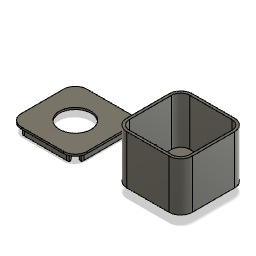
Case Button v3 (Autodesk Fusion 360 design; units mm, degrees)
Autodesk Fusion 360 part; units mm, degrees
sketch "Sketch1" plane through (0, 0, 0) normal (0, 1, 0) x (1, 0, 0)
  line L0 (5, 0) -> (23, 0)
  line L1 (28, -5) -> (28, -23)
  line L2 (23, -28) -> (5, -28)
  line L3 (0, -23) -> (0, -5)
  arc A0 (5, 0) -> (0, -5) centre (5, -5) ccw
  arc A1 (28, -5) -> (23, 0) centre (23, -5) ccw
  arc A2 (23, -28) -> (28, -23) centre (23, -23) ccw
  arc A3 (0, -23) -> (5, -28) centre (5, -23) ccw
  point P0 (28, 0)
  point P1 (0, -28)
  dimension "d1" = 28
  dimension "d2" = 28
  dimension "d3" = 5
  constraint horizontal L0
  constraint vertical L1
  constraint horizontal L2
  constraint vertical L3
  constraint coincident origin L0
  constraint coincident origin L3
  constraint tangent L0 A0
  constraint tangent L3 A0
  constraint coincident P0 L0
  constraint coincident P0 L1
  constraint tangent L0 A1
  constraint tangent L1 A1
  constraint equal A0 A1
  constraint tangent L1 A2
  constraint tangent L2 A2
  constraint equal A0 A2
  constraint coincident P1 L2
  constraint coincident P1 L3
  constraint tangent L2 A3
  constraint tangent L3 A3
  constraint equal A0 A3
  measures "d1" distance of origin P0
  measures "d2" distance of origin P1
  measures "d3" radius of A0
extrude "Extrude1" add sketch "Sketch1" along normal blind 0.8 makes body 1
sketch "Sketch2" plane through (0, 0.8, 0) normal (0, 1, 0) x (-1, 0, 0)
  arc A0 (-5, 0) -> (0, 5) centre (-5, 5) ccw
  line L0 (0, 5) -> (0, 23)
  arc A1 (0, 23) -> (-5, 28) centre (-5, 23) ccw
  line L1 (-5, 28) -> (-23, 28)
  arc A2 (-23, 28) -> (-28, 23) centre (-23, 23) ccw
  line L2 (-28, 23) -> (-28, 5)
  arc A3 (-28, 5) -> (-23, 0) centre (-23, 5) ccw
  line L3 (-23, 0) -> (-5, 0)
  line L4 (0, 14) -> (-28, 14)
  line L5 (-14, 0) -> (-14, 28)
  circle A4 centre (-14, 14) radius 6.75
  dimension "d6" = 13.5
  constraint midpoint L0 L4.start
  constraint midpoint L2 L4.end
  constraint midpoint L3 L5.start
  constraint midpoint L1 L5.end
  constraint midpoint L4 A4.centre
  measures "d6" diameter of A4
extrude "Extrude2" cut sketch "Sketch2" against normal blind 10 contours L4 L5 A4 | L4 L5 A4 | L4 L5 A4 | L4 L5 A4 bodies 1
sketch "Sketch3" plane through (0, 0, 0) normal (0, -1, 0) x (1, 0, 0)
  circle A0 centre (14, 14) radius 6.75
  arc A1 (0, 5) -> (5, 0) centre (5, 5) ccw
  line L0 (5, 0) -> (23, 0)
  arc A2 (23, 0) -> (28, 5) centre (23, 5) ccw
  line L1 (28, 5) -> (28, 23)
  arc A3 (28, 23) -> (23, 28) centre (23, 23) ccw
  line L2 (23, 28) -> (5, 28)
  arc A4 (5, 28) -> (0, 23) centre (5, 23) ccw
  line L3 (0, 23) -> (0, 5)
  arc A5 (5, 26.7) -> (1.3, 23) centre (5, 23) ccw
  line L4 (1.3, 23) -> (1.3, 5)
  arc A6 (1.3, 5) -> (5, 1.3) centre (5, 5) ccw
  line L5 (5, 1.3) -> (23, 1.3)
  arc A7 (23, 1.3) -> (26.7, 5) centre (23, 5) ccw
  line L6 (26.7, 5) -> (26.7, 23)
  arc A8 (26.7, 23) -> (23, 26.7) centre (23, 23) ccw
  line L7 (23, 26.7) -> (5, 26.7)
  arc A9 (5, 25.9) -> (2.1, 23) centre (5, 23) ccw
  line L8 (2.1, 23) -> (2.1, 5)
  arc A10 (2.1, 5) -> (5, 2.1) centre (5, 5) ccw
  line L9 (5, 2.1) -> (23, 2.1)
  arc A11 (23, 2.1) -> (25.9, 5) centre (23, 5) ccw
  line L10 (25.9, 5) -> (25.9, 23)
  arc A12 (25.9, 23) -> (23, 25.9) centre (23, 23) ccw
  line L11 (23, 25.9) -> (5, 25.9)
  dimension "d9" = -1.3
  dimension "d10" = -2.1
extrude "Extrude3" add sketch "Sketch3" along normal blind 3.2 contours A5 L4 A6 L5 A7 L6 A8 L7 bodies 1
sketch "Sketch4" plane through (0, 0.8, 0) normal (0, 1, 0) x (-1, 0, 0)
  circle A0 centre (-14, 14) radius 6.75
  arc A1 (-5, 0) -> (0, 5) centre (-5, 5) ccw
  line L0 (0, 5) -> (0, 23)
  arc A2 (0, 23) -> (-5, 28) centre (-5, 23) ccw
  line L1 (-5, 28) -> (-23, 28)
  arc A3 (-23, 28) -> (-28, 23) centre (-23, 23) ccw
  line L2 (-28, 23) -> (-28, 5)
  arc A4 (-28, 5) -> (-23, 0) centre (-23, 5) ccw
  line L3 (-23, 0) -> (-5, 0)
  line L4 (-50, 0) -> (-68, 0)
  line L5 (-73, 5) -> (-73, 23)
  line L6 (-68, 28) -> (-50, 28)
  line L7 (-45, 23) -> (-45, 5)
  arc A5 (-50, 0) -> (-45, 5) centre (-50, 5) ccw
  arc A6 (-73, 5) -> (-68, 0) centre (-68, 5) ccw
  arc A7 (-68, 28) -> (-73, 23) centre (-68, 23) ccw
  arc A8 (-45, 23) -> (-50, 28) centre (-50, 23) ccw
  point P0 (-45, 0)
  point P1 (-73, 0)
  point P2 (-45, 28)
  dimension "d13" = 28
  dimension "d14" = 28
  dimension "d15" = 5
  constraint horizontal L4
  constraint vertical L5
  constraint horizontal L6
  constraint vertical L7
  constraint coincident P0 L4
  constraint coincident P0 L7
  constraint tangent L4 A5
  constraint tangent L7 A5
  constraint coincident P1 L4
  constraint coincident P1 L5
  constraint tangent L4 A6
  constraint tangent L5 A6
  constraint equal A5 A6
  constraint tangent L5 A7
  constraint tangent L6 A7
  constraint equal A5 A7
  constraint coincident P2 L6
  constraint coincident P2 L7
  constraint tangent L6 A8
  constraint tangent L7 A8
  constraint equal A5 A8
  measures "d13" distance of P0 P1
  measures "d14" distance of P0 P2
  measures "d15" radius of A5
extrude "Extrude4" add sketch "Sketch4" along normal blind 0.8 separate body contours L4 L5 L6 L7 A5 A6 A7 A8 makes body 2
sketch "Sketch5" plane through (0, 1.6, 0) normal (0, 1, 0) x (-1, 0, 0)
  arc A0 (-50, 0) -> (-45, 5) centre (-50, 5) ccw
  line L0 (-45, 5) -> (-45, 23)
  arc A1 (-45, 23) -> (-50, 28) centre (-50, 23) ccw
  line L1 (-50, 28) -> (-68, 28)
  arc A2 (-68, 28) -> (-73, 23) centre (-68, 23) ccw
  line L2 (-73, 23) -> (-73, 5)
  arc A3 (-73, 5) -> (-68, 0) centre (-68, 5) ccw
  line L3 (-68, 0) -> (-50, 0)
  arc A4 (-46.1, 23) -> (-50, 26.9) centre (-50, 23) ccw
  line L4 (-50, 26.9) -> (-68, 26.9)
  arc A5 (-68, 26.9) -> (-71.9, 23) centre (-68, 23) ccw
  line L5 (-71.9, 23) -> (-71.9, 5)
  arc A6 (-71.9, 5) -> (-68, 1.1) centre (-68, 5) ccw
  line L6 (-68, 1.1) -> (-50, 1.1)
  arc A7 (-50, 1.1) -> (-46.1, 5) centre (-50, 5) ccw
  line L7 (-46.1, 5) -> (-46.1, 23)
  dimension "d18" = -1.1
extrude "Extrude5" add sketch "Sketch5" along normal blind 20 bodies 2
sketch "Sketch6" plane through (0, -3.2, 0) normal (0, -1, 0) x (1, 0, 0)
  line L0 (5, 25.9) -> (23, 25.9)
  arc A0 (25.9, 23) -> (23, 25.9) centre (23, 23) ccw
  line L1 (25.9, 23) -> (25.9, 5)
  arc A1 (23, 2.1) -> (25.9, 5) centre (23, 5) ccw
  line L2 (23, 2.1) -> (5, 2.1)
  arc A2 (2.1, 5) -> (5, 2.1) centre (5, 5) ccw
  line L3 (2.1, 5) -> (2.1, 23)
  arc A3 (5, 25.9) -> (2.1, 23) centre (5, 23) ccw
  line L4 (23, 26.7) -> (5, 26.7)
  arc A4 (5, 26.7) -> (1.3, 23) centre (5, 23) ccw
  line L5 (1.3, 23) -> (1.3, 5)
  arc A5 (1.3, 5) -> (5, 1.3) centre (5, 5) ccw
  line L6 (5, 1.3) -> (23, 1.3)
  arc A6 (23, 1.3) -> (26.7, 5) centre (23, 5) ccw
  line L7 (26.7, 5) -> (26.7, 23)
  arc A7 (26.7, 23) -> (23, 26.7) centre (23, 23) ccw
  line L8 (14, 25.9) -> (14, 1.3)
  line L9 (2.1, 14) -> (26.7, 14)
  line L10 (28.4207, 4.0183) -> (-0.4207, 4.0183)
  line L11 (-0.4207, 4.0183) -> (-0.4207, 23.9817)
  line L12 (-0.4207, 23.9817) -> (28.4207, 23.9817)
  line L13 (28.4207, 23.9817) -> (28.4207, 4.0183)
  line L14 (28.4207, 4.0183) -> (-0.4207, 23.9817) construction
  line L15 (-0.4207, 4.0183) -> (28.4207, 23.9817) construction
  line L16 (24, 1) -> (4, 1)
  line L17 (4, 1) -> (4, 27)
  line L18 (4, 27) -> (24, 27)
  line L19 (24, 27) -> (24, 1)
  line L20 (24, 1) -> (4, 27) construction
  line L21 (4, 1) -> (24, 27) construction
  point P0 (14, 14)
  point P1 (14, 14)
  constraint midpoint L0 L8.start
  constraint midpoint L6 L8.end
  constraint midpoint L3 L9.start
  constraint midpoint L7 L9.end
  constraint horizontal L10
  constraint perpendicular L10 L11
  constraint parallel L10 L12
  constraint parallel L11 L13
  constraint coincident L14 P1
  constraint coincident L15 P1
  constraint coincident L8 P1
  constraint coincident L9 P1
  constraint horizontal L16
  constraint perpendicular L16 L17
  constraint parallel L16 L18
  constraint parallel L17 L19
  constraint coincident L20 P1
  constraint coincident L21 P1
  constraint coincident P1 P0
extrude "Extrude6" cut sketch "Sketch6" against normal blind 3 contours A3 A4 L12 L17 | A0 A7 L12 L19 | A2 A5 L10 L17 | A1 A6 L10 L19 bodies 1
sketch "Sketch7" plane through (45, 0, 0) normal (-1, 0, 0) x (0, 0, 1)
  line L0 (5, 0.8) -> (23, 0.8)
  line L1 (23, 0.8) -> (23, 21.6)
  line L2 (23, 21.6) -> (5, 21.6)
  line L3 (5, 21.6) -> (5, 0.8)
  line L4 (14, 21.6) -> (14, 0.8)
  line L5 (16.5, 3.6782) -> (11.5, 3.6782)
  line L6 (11.5, 3.6782) -> (11.5, 6.6782)
  line L7 (11.5, 6.6782) -> (16.5, 6.6782)
  line L8 (16.5, 6.6782) -> (16.5, 3.6782)
  line L9 (16.5, 3.6782) -> (11.5, 6.6782) construction
  line L10 (11.5, 3.6782) -> (16.5, 6.6782) construction
  point P0 (14, 5.1782)
  dimension "d23" = 5
  dimension "d24" = 3
  constraint midpoint L2 L4.start
  constraint midpoint L0 L4.end
  constraint horizontal L5
  constraint perpendicular L5 L6
  constraint parallel L5 L7
  constraint parallel L6 L8
  constraint coincident L9 P0
  constraint coincident L10 P0
  constraint coincident L4 P0
  measures "d23" distance of L6.end L7.end
  measures "d24" distance of L5.end L6.end
extrude "Extrude7" cut sketch "Sketch7" against normal blind 4 contours L4 L5 L6 L7 | L4 L5 L7 L8 bodies 2
sketch "Sketch8" plane through (0, 1.6, 0) normal (0, 1, 0) x (-1, 0, 0)
  arc A0 (-46.1, 23) -> (-50, 26.9) centre (-50, 23) ccw
  line L0 (-50, 26.9) -> (-68, 26.9)
  arc A1 (-68, 26.9) -> (-71.9, 23) centre (-68, 23) ccw
  line L1 (-71.9, 23) -> (-71.9, 5)
  arc A2 (-71.9, 5) -> (-68, 1.1) centre (-68, 5) ccw
  line L2 (-68, 1.1) -> (-50, 1.1)
  arc A3 (-50, 1.1) -> (-46.1, 5) centre (-50, 5) ccw
  line L3 (-46.1, 5) -> (-46.1, 23)
  line L4 (-49.9308, 14.1272) -> (-54.2473, 16.1679)
  line L5 (-54.2473, 16.1679) -> (-54.1128, 12.4316)
  line L6 (-54.1128, 12.4316) -> (-49.9308, 14.1272)
  point P0 (-52.32, 13.6169)
extrude "Extrude8" cut sketch "Sketch8" against normal blind 0.2 contours L4 L5 L6 bodies 2
chamfer "Chamfer1" distance 0.4 angle 45 12 edges at (14, -3.2, 25.9) (23.5078, -3.2, 25.8552) (4.4922, -3.2, 25.8552) (2.1, -3.2, 14) (2.1431, -3.2, 23.4983) (2.1431, -3.2, 4.5017) (25.9, -3.2, 14) (25.8569, -3.2, 4.5017) (25.8569, -3.2, 23.4983) (14, -3.2, 2.1) (4.4922, -3.2, 2.1448) (23.5078, -3.2, 2.1448) on bodies 1
copy_body "Body->Comp1" bodies 1 removing the originals makes body 3 in component "Penutup atas"
copy_body "Body->Comp2" bodies 2 removing the originals makes body 4 in component "Body bawah"
component "Penutup atas" placed x (1, 0, 0) y (0, 1, 0) z (0, 0, 1) at (0, 0, 0)
component "Body bawah" placed x (1, 0, 0) y (0, 1, 0) z (0, 0, 1) at (0, 0, 0)
equation "d10 = -1.3 mm - 0.8 mm"
equation "d18 = -1 mm - 0.1 mm"
